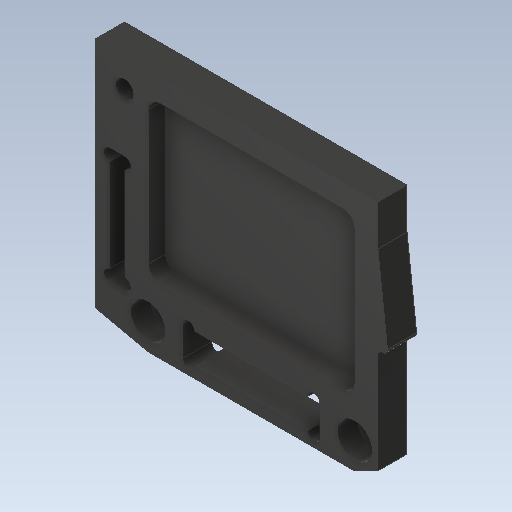
# Autodesk Inventor part: コックピット_サブフレーム_1_5_MIR
Saved by Autodesk Inventor 2020 (Build 240168000, 168)
## iProperties
Created: 2018-10-12
Part Number: コックピット_サブフレーム_1_5_MIR
Material: アセタール樹脂、黒
Document SubType Name: Modeling
Designer: taka
Density: 1.425 g/cm^3
Appearance: 滑らか - 黒
Author: taka
Autodesk Inventor part; units mm, degrees
ref_plane "YZ Plane" through (0, 0, 0) normal (1, 0, 0) x (0, 1, 0)
ref_plane "XZ Plane" through (0, 0, 0) normal (0, 1, 0) x (-1, 0, 0)
ref_plane "XY Plane" through (0, 0, 0) normal (0, 0, 1) x (1, 0, 0)
sketch "スケッチ1" plane through (0, 0, 0) normal (0, 0, 1) x (1, 0, 0)
  line L0 (-24.25, -20) -> (24.25, -20) construction
  line L1 (24.25, -20) -> (24.25, 20)
  line L2 (24.25, 20) -> (-24.25, 20)
  line L3 (-24.25, 20) -> (-24.25, -20)
  line L4 (-24.25, -20) -> (24.25, 20) construction
  line L5 (24.25, -20) -> (-24.25, 20) construction
  circle A0 centre (-15.25, -17.5) radius 1.55
  circle A1 centre (20.25, -17.5) radius 1.55
  line L6 (-9.25, -15) -> (14.25, -15) construction
  line L7 (14.25, -15) -> (14.25, -20) construction
  line L8 (14.25, -20) -> (-9.25, -20) construction
  line L9 (-9.25, -20) -> (-9.25, -15) construction
  line L10 (-24.25, -20) -> (-15.25, -22)
  line L11 (-15.25, -22) -> (20.25, -22)
  line L12 (20.25, -22) -> (24.25, -20)
  line L13 (14.3, -14.95) -> (-9.3, -14.95)
  line L14 (-9.3, -14.95) -> (-9.3, -20.05)
  line L15 (-9.3, -20.05) -> (14.3, -20.05)
  line L16 (14.3, -20.05) -> (14.3, -14.95)
  circle A2 centre (-8.25, -14.95) radius 1.05
  circle A3 centre (-8.25, -20.05) radius 1.05
  circle A4 centre (13.25, -14.95) radius 1.05
  circle A5 centre (13.25, -20.05) radius 1.05
  circle A6 centre (-19.25, 15) radius 1.55
  line L17 (-21.8, 5.05) -> (-19.2, 5.05)
  line L18 (-19.2, 5.05) -> (-19.2, -15.05)
  line L19 (-19.2, -15.05) -> (-21.8, -15.05)
  line L20 (-21.8, -15.05) -> (-21.8, 5.05)
  line L21 (-19.25, 5) -> (-21.75, 5) construction
  line L22 (-21.75, 5) -> (-21.75, -15) construction
  line L23 (-21.75, -15) -> (-19.25, -15) construction
  line L24 (-19.25, -15) -> (-19.25, 5) construction
  line L25 (2.5, -14.95) -> (2.5, -20.05) construction
  circle A7 centre (-21.8, 4) radius 1.05
  circle A8 centre (-19.2, 4) radius 1.05
  circle A9 centre (-21.8, -14) radius 1.05
  circle A10 centre (-19.2, -14) radius 1.05
  point P0 (0, 0)
  point P1 (0, 0)
  point P2 (-9.25, -17.5)
  dimension "d8" = 2.1
  dimension "d22" = 2.1
  dimension "d1" = 5
  dimension "d2" = 3.1
  dimension "d3" = 35.5
  dimension "d4" = 2
  dimension "d5" = 40
  dimension "d6" = 23.5
  dimension "d7" = 0.05
  dimension "d9" = 3.1
  dimension "d10" = 5
  dimension "d11" = 5
  dimension "d12" = 0.05
  dimension "d13" = 17.75
  dimension "d14" = 48.5
  dimension "d15" = 4
  dimension "d18" = 2.5
  dimension "d19" = 2.5
  dimension "d20" = 5
  dimension "d21" = 15
  dimension "d23" = 25
  constraints: 52 end point, 10 parallel, 8 point on line, 6 horizontal alignment, 6 vertical alignment, 5 midpoint, 5 perpendicular, 3 centre point, 3 horizontal, 1 collinear, 1 equal radius, 22 other
  measures "d1" distance of L8.end L6.start
  measures "d2" diameter of A0
  measures "d3" distance of A1.centre A0.centre
  measures "d4" distance between parallel lines of L11 L0
  measures "d5" distance of L0.end L1.end
  measures "d6" distance of L6.start L6.end
  measures "d7" distance between parallel lines of L13 L6
  measures "d9" diameter of A6
  measures "d10" distance from line of L3 A6.centre
  measures "d11" distance from line of L2 A6.centre
  measures "d12" distance between parallel lines of L17 L21
  measures "d13" distance from line of A0.centre L25
  measures "d14" distance of L1.end L2.end
  measures "d15" distance from line of L1 A1.centre
  measures "d18" distance of L21.start L21.end
  measures "d19" distance between parallel lines of L22 L3
  measures "d20" distance between parallel lines of L23 L0
  measures "d21" distance between parallel lines of L2 L21
  measures "d23" distance between parallel lines of L21 L0
extrude "押し出し1" add sketch "スケッチ1" along normal blind 5
sketch "スケッチ3" plane through (0, 0, 5) normal (0, 0, 1) x (1, 0, 0)
  line L0 (-15.2, 16) -> (20.25, 16)
  line L1 (20.25, 16) -> (20.25, -10.95)
  line L2 (20.25, -10.95) -> (-15.2, -10.95)
  line L3 (-15.2, -10.95) -> (-15.2, 16)
  line L4 (24.25, -20) -> (24.25, 20) projected
  line L5 (24.25, 20) -> (-24.25, 20) projected
  line L6 (-7.2, -14.95) -> (12.2, -14.95) projected
  line L7 (-19.2, 2.95) -> (-19.2, -12.95) projected
  point P0 (0, 0)
  dimension "d26" = 4
  dimension "d27" = 4
  dimension "d28" = 4
  dimension "d29" = 4
  constraints: 8 end point, 2 parallel, 1 horizontal, 1 perpendicular
  measures "d26" distance between parallel lines of L1 L4
  measures "d27" distance between parallel lines of L5 L0
  measures "d28" distance between parallel lines of L6 L2
  measures "d29" distance between parallel lines of L3 L7
extrude "押し出し2" cut sketch "スケッチ3" against normal blind 3
sketch "スケッチ4" plane through (0, 0, 5) normal (0, 0, 1) x (1, 0, 0)
  circle A0 centre (-15.25, -17.5) radius 3
  circle A1 centre (20.25, -17.5) radius 3
  circle A2 centre (-15.25, -17.5) radius 1.55 projected
  circle A3 centre (20.25, -17.5) radius 1.55 projected
  point P0 (0, 0)
  dimension "d32" = 6
  dimension "d33" = 6
  constraints: 2 centre point, 2 concentric
  measures "d32" diameter of A1
  measures "d33" diameter of A0
extrude "押し出し3" cut sketch "スケッチ4" against normal blind 3.5
fillet "フィレット1" radius 2 4 edges at (-15.2, 16, 3.5) (-15.2, -10.95, 3.5) (20.25, -10.95, 3.5) (20.25, 16, 3.5)
sketch "スケッチ10" plane through (24.25, -20, 0) normal (1, 0, 0) x (0, 0, -1)
  line L0 (-5, 40) -> (-5, 0) projected
  line L1 (-5, 33) -> (0, 33)
  line L2 (0, 33) -> (0, 18)
  line L3 (0, 18) -> (-5, 18)
  line L4 (-5, 18) -> (-5, 33)
  line L5 (0, 40) -> (-5, 40) projected
  point P0 (0, 20)
  dimension "d52" = 5
  dimension "d53" = 15
  dimension "d54" = 7
  constraints: 8 end point, 2 parallel, 1 horizontal, 1 perpendicular, 1 point on line
  measures "d52" distance of L2.end L3.end
  measures "d53" distance of L1.end L2.end
  measures "d54" distance between parallel lines of L1 L5
extrude "押し出し9" add sketch "スケッチ10" along normal blind 1.75
sketch "スケッチ11" plane through (0, 0, 0) normal (0, 0, -1) x (-1, 0, 0)
  line L0 (-24.25, -2) -> (-26, -2) projected
  line L1 (-26, -2) -> (-26, 13)
  line L2 (-24.25, 13) -> (-24.25, 20) projected
  line L3 (-26, 13) -> (-24.25, 13)
  line L4 (-26, -2) -> (-26, 13) projected
  line L5 (-24.25, 13) -> (-26, -2)
  point P0 (0, 0)
  constraints: 6 end point, 1 perpendicular, 1 vertical
extrude "押し出し10" cut sketch "スケッチ11" against normal through all
fillet "フィレット2" radius 0.8 1 edges at (26, -2, 2.5)
fillet "フィレット3" radius 0.5 1 edges at (24.25, -2, 2.5)
equation "\"d11\" = d10"
equation "\"d13\" = 0.5 * d3"
equation "\"d27\" = d26"
equation "\"d28\" = d26"
equation "\"d29\" = d26"
